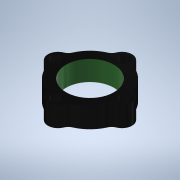
# Autodesk Inventor part: Knee_clamp
Saved by Autodesk Inventor 2022 (Build 260153000, 153)
## iProperties
Part Number: Knee_clamp
Material: アルミニウム 2014-T4
Document SubType Name: Modeling
Designer: Masato Kubotera
Density: 2.8 g/cm^3
Appearance: Smooth - Black
Mass: 1.74204 g
Surface Area: 9.17131 cm^2
Volume: 0.622156 cm^3
Description: A2017 T5
Author: Masato Kubotera
Revision Number: Rev.2 Specifications for RoboCup 2023: Anodized aluminum staining process added.
Autodesk Inventor part; units mm, degrees
ref_plane "YZ Plane" through (0, 0, 0) normal (1, 0, 0) x (0, 1, 0)
ref_plane "XZ Plane" through (0, 0, 0) normal (0, 1, 0) x (-1, 0, 0)
ref_plane "XY Plane" through (0, 0, 0) normal (0, 0, 1) x (1, 0, 0)
sketch "スケッチ1" plane through (0, 0, 0) normal (0, 0, 1) x (1, 0, 0)
  circle A0 centre (0, 0) radius 5.985
  circle A1 centre (0, 8.5) radius 1.35
  line L0 (0, 8.5) -> (0, 0) construction
  circle A2 centre (0, 0) radius 8.5 construction
  circle A3 centre (0, 0) radius 10.5 construction
  arc A4 (2.5, 8.124) -> (-2.5, 8.124) centre (0, 7.9968) ccw
  arc A5 (-8.124, 2.5) -> (-8.124, -2.5) centre (-7.9968, 0) ccw
  circle A6 centre (-8.5, 0) radius 1.35
  arc A7 (-2.5, -8.124) -> (2.5, -8.124) centre (0, -7.9968) ccw
  circle A8 centre (0, -8.5) radius 1.35
  arc A9 (8.124, -2.5) -> (8.124, 2.5) centre (7.9968, 0) ccw
  circle A10 centre (8.5, 0) radius 1.35
  arc A11 (-2.5, 8.124) -> (-8.124, 2.5) centre (0, 0) ccw
  arc A12 (-8.124, -2.5) -> (-2.5, -8.124) centre (0, 0) ccw
  arc A13 (2.5, -8.124) -> (8.124, -2.5) centre (0, 0) ccw
  arc A14 (8.124, 2.5) -> (2.5, 8.124) centre (0, 0) ccw
  point P0 (0, 10.5)
  point P1 (-10.5, 0)
  point P2 (0, -10.5)
  point P3 (10.5, 0)
  dimension "d39" = 21
  dimension "d1" = 11.97
  dimension "d2" = 2.7
  dimension "d5" = 17
  dimension "d40" = 5
  dimension "d43" = 360
  constraints: 20 point on circle, 14 centre point, 8 coincident, 2 end point, 2 vertical alignment, 1 point on line, 1 vertical, 31 other
  measures "d1" diameter of A0
  measures "d2" diameter of A1
  measures "d5" diameter of A2
  measures "d40" distance of A4.start A2.end
extrude "押し出し1" add sketch "スケッチ1" along normal blind 5
fillet "フィレット1" radius 2 8 edges at (-8.124, -2.5, 2.5) (-2.5, -8.124, 2.5) (2.5, -8.124, 2.5) (8.124, -2.5, 2.5) (8.124, 2.5, 2.5) (2.5, 8.124, 2.5) (-2.5, 8.124, 2.5) (-8.124, 2.5, 2.5)
